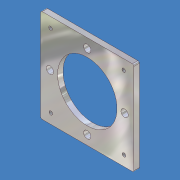
# Autodesk Inventor part: BB2-InterfacePlate
Saved by Autodesk Inventor 2012 (Build 160160000, 160)
## iProperties
Company: FirstCadLibrary
Shininess: 64.0
Length Units: 11269
Angle Units: 11279
Time Units: 11290
Mass Units: 11283
Length Display Precision: 3
Angle Display Precision: 2
Compacted: True
Part Number: BB2-InterfacePlate
Document SubType Name: Modeling
Created: 2007-01-08
Material: Aluminum-6061
Designer: Ed Sparks
Catalog Web Link: www.banebots.com
Vendor: BaneBots
Mass: 26.5594 g
Surface Area: 70.4801 cm^2
Volume: 9.80051 cm^3
Density: 2.71 g/cm^3
Density: 0.0
Volumn: 0.0
Area: 0.0
PropertySet Name: Model Information
Control State: 0
Master: False
Checked Out: False
Author: Ed Sparks
Autodesk Inventor part; units mm, degrees
ref_plane "YZ Plane" through (0, 0, 0) normal (1, 0, 0) x (0, 1, 0)
ref_plane "XZ Plane" through (0, 0, 0) normal (0, 1, 0) x (-1, 0, 0)
ref_plane "XY Plane" through (0, 0, 0) normal (0, 0, 1) x (1, 0, 0)
sketch "Sketch1" plane through (0, 0, 0) normal (0, 0, 1) x (1, 0, 0)
  line L0 (-31.75, 31.75) -> (31.75, 31.75)
  line L1 (31.75, 31.75) -> (31.75, -31.75)
  line L2 (31.75, -31.75) -> (-31.75, -31.75)
  line L3 (-31.75, -31.75) -> (-31.75, 31.75)
  line L4 (0, 0) -> (31.75, 0) construction
  line L5 (0, 0) -> (-31.75, 0) construction
  line L6 (0, 0) -> (0, 31.75) construction
  line L7 (0, 0) -> (0, -31.75) construction
  dimension "d0" = 63.5
  dimension "d1" = 63.5
  constraints: 16 end point, 4 midpoint, 2 collinear, 2 parallel, 1 horizontal, 1 perpendicular, 1 other
  measures "d0" distance of L0.start L0.end
  measures "d1" distance of L0.end L1.end
extrude "Extrusion1" add sketch "Sketch1" along normal mid plane 3.7
sketch "Sketch2" plane through (0, 0, 1.85) normal (0, 0, 1) x (1, 0, 0)
  point P0 (0, 0)
hole "Hole1" at (0, 0, 1.85) direction (0, 0, -1) diameter 40.45 end through all
sketch "Sketch3" plane through (0, 0, 1.85) normal (0, 0, 1) x (1, 0, 0)
  circle A0 centre (0, 0) radius 20.225 projected
  point P0 (0, 25.4)
  dimension "d11" = 25.4
  constraints: 1 vertical alignment
  measures "d11" distance of point (0, 25.4) A0.centre
hole "Hole2" at (0, 25.4, 1.85) direction (0, 0, -1) diameter 5 end through all
pattern_circular "Circular Pattern1" count 4 over 360 about axis through (0, 0, -88.0288) along (0, 0, 1) of "Hole2"
sketch "Sketch4" plane through (0, 0, 1.85) normal (0, 0, 1) x (1, 0, 0)
  circle A0 centre (-25.4, 0) radius 2.5 projected
  circle A1 centre (0, 25.4) radius 2.5 projected
  point P0 (-25, 24.8272)
  dimension "d24" = 24.8272
  dimension "d25" = 25
  measures "d24" vertical distance of A0.centre point (-25, 24.827)
  measures "d25" horizontal distance of A1.centre point (-25, 24.827)
hole "Hole3" at (-25, 24.8272, 1.85) direction (0, 0, -1) diameter 2.459 end through all thread size "M3x0.5" class "6H" standard "ANSI Metric M Profile"
pattern_circular "Circular Pattern2" count 4 over 360 about axis through (0, 0, -88.0288) along (0, 0, 1) of "Hole3"
fillet "Fillet1" radius 1 4 edges at (-31.75, 31.75, 0) (-31.75, -31.75, 0) (31.75, -31.75, 0) (31.75, 31.75, 0)
body "Solid1"
